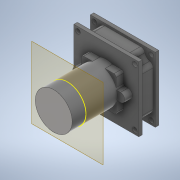
# Autodesk Inventor part: e-CAM50_CUNX
Saved by Autodesk Inventor 2020.4 (Build 244396000, 396)
## iProperties
Part Number: e-CAM50_CUNX
Material: 一般
Document SubType Name: Modeling
Designer: Masato Kubotera
Density: 0.854732 g/cm^3
Appearance: 滑らか - 黒
Mass: 10.8 g
Surface Area: 43.4114 cm^2
Volume: 12.6355 cm^3
Catalog Web Link: https://www.shikino.co.jp/products/product-kbcr-s02mu.php
Description: ReadyMade
Author: Masato Kubotera
Autodesk Inventor part; units mm, degrees
ref_plane "YZ Plane" through (0, 0, 0) normal (1, 0, 0) x (0, 1, 0)
ref_plane "XZ Plane" through (0, 0, 0) normal (0, 1, 0) x (-1, 0, 0)
ref_plane "XY Plane" through (0, 0, 0) normal (0, 0, 1) x (1, 0, 0)
sketch "スケッチ1" plane through (0, 0, 0) normal (0, 0, 1) x (1, 0, 0)
  line L0 (15, 15) -> (-15, 15)
  line L1 (-15, 15) -> (-15, -15)
  line L2 (-15, -15) -> (15, -15)
  line L3 (15, -15) -> (15, 15)
  line L4 (15, 15) -> (-15, -15) construction
  line L5 (-15, 15) -> (15, -15) construction
  line L6 (-13.14, 13.14) -> (13.14, 13.14) construction
  line L7 (13.14, 13.14) -> (13.14, -13.14) construction
  line L8 (13.14, -13.14) -> (-13.14, -13.14) construction
  line L9 (-13.14, -13.14) -> (-13.14, 13.14) construction
  line L10 (-13.14, 13.14) -> (13.14, -13.14) construction
  line L11 (13.14, 13.14) -> (-13.14, -13.14) construction
  circle A0 centre (-13.14, -13.14) radius 1.1
  line L12 (-15, 0) -> (15, 0) construction
  line L13 (0, 15) -> (0, -15) construction
  circle A1 centre (-13.14, 13.14) radius 1.1
  circle A2 centre (13.14, -13.14) radius 1.1
  circle A3 centre (13.14, 13.14) radius 1.1
  circle A4 centre (-13.14, -13.14) radius 2 construction
  circle A5 centre (-13.14, 13.14) radius 2 construction
  circle A6 centre (13.14, -13.14) radius 2 construction
  circle A7 centre (13.14, 13.14) radius 2 construction
  circle A8 centre (0, 0) radius 8.5
  line L14 (-7, 8) -> (7, 8)
  line L15 (8, 7) -> (8, -7)
  line L16 (7, -8) -> (-7, -8)
  line L17 (-8, -7) -> (-8, 7)
  line L18 (-8, 8) -> (8, -8) construction
  line L19 (8, 8) -> (-8, -8) construction
  arc A9 (-7, 8) -> (-8, 7) centre (-7, 7) ccw
  arc A10 (-8, -7) -> (-7, -8) centre (-7, -7) ccw
  arc A11 (7, -8) -> (8, -7) centre (7, -7) ccw
  arc A12 (8, 7) -> (7, 8) centre (7, 7) ccw
  arc A13 (-10, 2) -> (-10, -2) centre (-10, 0) ccw
  line L20 (-10, 2) -> (-8, 2)
  line L21 (-10, -2) -> (-8, -2)
  arc A14 (10, -2) -> (10, 2) centre (10, 0) ccw
  line L22 (10, 2) -> (8, 2)
  line L23 (10, -2) -> (8, -2)
  line L24 (-8.2717, 14) -> (8.2717, 14)
  line L25 (14, 8.2717) -> (14, -8.2717)
  line L26 (8.2717, -14) -> (-8.2717, -14)
  line L27 (-14, -8.2717) -> (-14, 8.2717)
  line L28 (-14, 14) -> (14, -14) construction
  line L29 (14, 14) -> (-14, -14) construction
  arc A15 (12.456, -10.219) -> (10.219, -12.456) centre (13.14, -13.14) ccw
  arc A16 (-10.219, -12.456) -> (-12.456, -10.219) centre (-13.14, -13.14) ccw
  arc A17 (10.219, 12.456) -> (12.456, 10.219) centre (13.14, 13.14) ccw
  arc A18 (-12.456, 10.219) -> (-10.219, 12.456) centre (-13.14, 13.14) ccw
  arc A19 (8.2717, -14) -> (10.219, -12.456) centre (8.2717, -12) ccw
  arc A20 (12.456, -10.219) -> (14, -8.2717) centre (12, -8.2717) ccw
  arc A21 (14, 8.2717) -> (12.456, 10.219) centre (12, 8.2717) ccw
  arc A22 (10.219, 12.456) -> (8.2717, 14) centre (8.2717, 12) ccw
  arc A23 (-8.2717, 14) -> (-10.219, 12.456) centre (-8.2717, 12) ccw
  arc A24 (-12.456, 10.219) -> (-14, 8.2717) centre (-12, 8.2717) ccw
  arc A25 (-14, -8.2717) -> (-12.456, -10.219) centre (-12, -8.2717) ccw
  arc A26 (-10.219, -12.456) -> (-8.2717, -14) centre (-8.2717, -12) ccw
  point P0 (8, 2)
  point P1 (8, -2)
  point P2 (14, -10.2659)
  point P3 (10.2659, -14)
  point P4 (-14, -10.2659)
  point P5 (-10.2659, -14)
  point P6 (14, 10.2659)
  point P7 (10.2659, 14)
  point P8 (-14, 10.2659)
  point P9 (-10.2659, 14)
  dimension "d0" = 30
  dimension "d1" = 30
  dimension "d5" = 2.2
  dimension "d6" = 4
  dimension "d40" = 26.28
  dimension "d41" = 26.28
  dimension "d42" = 17
  dimension "d43" = 16
  dimension "d44" = 16
  dimension "d57" = 1
  dimension "d58" = 2
  dimension "d60" = 20
  dimension "d65" = 2
  dimension "d66" = 3
  dimension "d67" = 1
  constraints: 61 end point, 44 point on circle, 27 centre point, 27 point on line, 25 tangent, 20 symmetric about line, 14 midpoint, 10 equal radius, 9 parallel, 6 perpendicular, 4 coincident, 4 horizontal, 11 other
  measures "d0" distance of L2.end L4.end
  measures "d1" distance of L1.start L4.end
  measures "d5" diameter of A0
  measures "d6" diameter of A4
  measures "d40" distance of L7.end L8.end
  measures "d41" distance of L8.end L6.start
  measures "d42" diameter of A8
  measures "d43" distance of L18.end L19.end
  measures "d44" distance of L19.start L18.end
  measures "d57" radius of A9
  measures "d58" radius of A13
  measures "d60" distance of A14.centre A13.centre
  measures "d65" radius of A19
  measures "d66" radius of A15
  measures "d67" distance between parallel lines of L2 L26
extrude "押し出し1" add sketch "スケッチ1" along normal blind 9.2 contours L3 L2 L1 L0 | A8 L23 L15 L22 | A8 L22 A14 L23 | L22 L15 A8 | A8 L15 L23 | L15 A8 L16 L17 L14 | A8 L14 A12 L15 | L15 A11 L16 A8 | L14 A8 | A8 L16 | A8 L17 A9 L14 | L16 A10 L17 A8 | L17 L20 A8 | A8 L21 L17 | L20 L17 L21 A8 | A8 L21 A13 L20 | L24 A22 A17 A21 L25 A20 A15 A19 L26 A26 A16 A25 L27 A24 A18 A23
extrude "押し出し2" cut sketch "スケッチ1" along normal blind 7.6 contours L3 L2 L1 L0
extrude "押し出し3" add sketch "スケッチ1" along normal blind 1.6 contours L3 L2 L1 L0 | A8 L23 L15 L22 | A8 L22 A14 L23 | L22 L15 A8 | A8 L15 L23 | L15 A8 L16 L17 L14 | A8 L14 A12 L15 | L15 A11 L16 A8 | L14 A8 | A8 L16 | A8 L17 A9 L14 | L16 A10 L17 A8 | L17 L20 A8 | A8 L21 L17 | L20 L17 L21 A8 | A8 L21 A13 L20 | L24 A22 A17 A21 L25 A20 A15 A19 L26 A26 A16 A25 L27 A24 A18 A23
extrude "押し出し4" add sketch "スケッチ1" along normal blind 12.7 contours A8 L23 L15 L22 | A8 L22 A14 L23 | A8 L14 A12 L15 | L15 A11 L16 A8 | A8 L17 A9 L14 | L16 A10 L17 A8 | L20 L17 L21 A8 | A8 L21 A13 L20
extrude "押し出し5" add sketch "スケッチ1" along normal blind 33.5 contours A8 L23 L15 L22 | L22 L15 A8 | A8 L15 L23 | L15 A8 L16 L17 L14 | L14 A8 | A8 L16 | L17 L20 A8 | A8 L21 L17 | L20 L17 L21 A8
ref_plane "作業平面1" through (0, 0, 27.2) normal (0, 0, 1) x (1, 0, 0)
sketch "スケッチ2" plane through (0, 0, 27.2) normal (0, 0, 1) x (1, 0, 0)
  circle A0 centre (0, 0) radius 8.5 projected
  line L0 (-8.5, 0) -> (8.5, 0)
  arc A1 (8.2614, -2) -> (8.2614, 2) centre (0, 0) ccw projected
  arc A2 (2.8723, 8) -> (-2.8723, 8) centre (0, 0) ccw projected
  line L1 (0, 8.5) -> (0, -8.5)
  constraints: 4 end point, 4 point on circle, 2 midpoint, 1 coincident, 1 horizontal, 1 perpendicular
equation "\"d40\" = d41"
equation "\"d44\" = d43"
